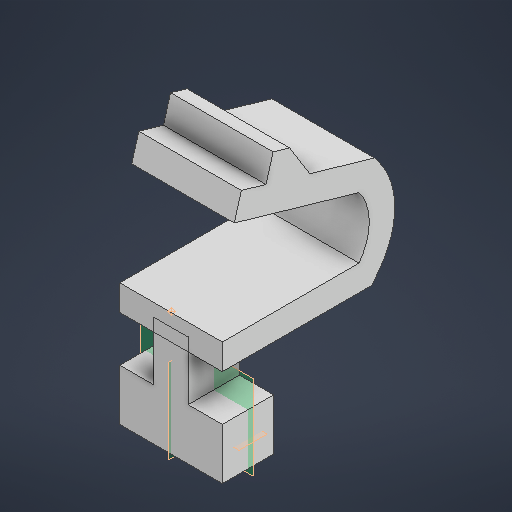
# Autodesk Inventor part: Clipper
Saved by Autodesk Inventor 2027 (Build 310192000, 192)
## iProperties
Created: 2026-03-31
Part Number: Clipper
Material: Generisch
Document SubType Name: Modeling
Designer: thomas
Density: 1 g/cm^3
Appearance: Vorgabe
Author: thomas
Autodesk Inventor part; units mm, degrees
ref_plane "YZ Plane" through (0, 0, 0) normal (1, 0, 0) x (0, 1, 0)
ref_plane "XZ Plane" through (0, 0, 0) normal (0, 1, 0) x (-1, 0, 0)
ref_plane "XY Plane" through (0, 0, 0) normal (0, 0, 1) x (1, 0, 0)
sketch "Sketch6" plane through (0, 0, 0) normal (0, 0, 1) x (1, 0, 0)
  line L0 (3, -1.5) -> (3, 1.5)
  line L1 (3, 1.5) -> (-3, 1.5)
  line L2 (-3, 1.5) -> (-3, -1.5)
  line L3 (-3, -1.5) -> (3, -1.5)
  line L4 (3, -1.5) -> (-3, 1.5) construction
  line L5 (3, 1.5) -> (-3, -1.5) construction
  point P0 (0, 0)
  dimension "d11" = 3
  dimension "d12" = 6
  constraints: 12 end point, 2 midpoint, 2 parallel, 1 perpendicular, 1 vertical
  measures "d11" distance of L0.start L0.end
  measures "d12" distance of L1.end L0.end
extrude "Extrusion4" add sketch "Sketch6" along normal mid plane 3
ref_plane "Work Plane1" through (0, 0, 0) normal (0, 0, 1) x (1, 0, 0)
sketch "Sketch8" plane through (0, 0, 1.5) normal (0, 0, 1) x (1, 0, 0)
  line L0 (-1, -1.5) -> (-1, 1.5)
  line L1 (-1, 1.5) -> (1, 1.5)
  line L2 (1, 1.5) -> (1, -1.5)
  line L3 (1, -1.5) -> (-1, -1.5)
  line L4 (-1, -1.5) -> (1, 1.5) construction
  line L5 (-1, 1.5) -> (1, -1.5) construction
  line L6 (3, 1.5) -> (-3, 1.5) projected
  point P0 (0, 0)
  dimension "d19" = 3
  dimension "d20" = 2
  constraints: 12 end point, 2 midpoint, 2 parallel, 1 collinear, 1 perpendicular
  measures "d19" distance of L0.start L0.end
  measures "d20" distance of L0.end L1.end
extrude "Extrusion6" add sketch "Sketch8" along normal blind 1.5
ref_plane "Work Plane4" through (-3, 0, -1.5) normal (0, 1, 0) x (1, 0, 0)
ref_plane "Work Plane5" through (0, -1.5, 1.5) normal (-1, 0, 0) x (0, 0, 1)
sketch "Sketch9" plane through (0, 0, 3) normal (0, 0, 1) x (1, 0, 0)
  point P0 (0, 0)
sketch "Sketch10" plane through (0, -1.5, 1.5) normal (-1, 0, 0) x (0, 0, 1)
  point P0 (-1.5, 1.5)
sketch "Sketch11" plane through (0, 0, 3) normal (0, 0, 1) x (1, 0, 0)
  point P0 (0, 0)
sketch "Sketch12" plane through (0, -1.5, 1.5) normal (-1, 0, 0) x (0, 0, 1)
  point P0 (-1.5, 1.5)
sketch "Sketch13" plane through (0, -1.5, 1.5) normal (-1, 0, 0) x (0, 0, 1)
  point P0 (-1.5, 1.5)
sketch "Sketch15" plane through (0, -1.5, 1.5) normal (-1, 0, 0) x (0, 0, 1)
  line L0 (4.175, 0) -> (4.175, 8)
  arc A0 (7.75, 8) -> (4.175, 8) centre (5.9625, 5.5907) ccw
  line L1 (7.75, 8) -> (9.858, 0.6982)
  line L2 (0, 0) -> (1.5, 0) projected
  line L3 (1.5, 0) -> (6.1638, 0) construction
  line L4 (1.5, 3) -> (1.5, 0) projected
  point P0 (-1.5, 1.5)
  dimension "d31" = 8
  dimension "d34" = 7.6
  dimension "d41" = 2.675
  dimension "d48" = 3.575
  constraints: 6 end point, 2 point on circle, 1 centre point, 1 horizontal, 1 point on line, 1 vertical
  measures "d31" distance of L0.start L0.end
  measures "d34" distance of L1.start L1.end
  measures "d41" distance between parallel lines of L0 L4
  measures "d48" distance of L1.start L0.end
sketch "Sketch18" plane through (-3, -1.5, -1.5) normal (0, -1, 0) x (1, 0, 0)
  line L0 (6, 5.675) -> (0, 5.675)
  line L1 (0, 5.675) -> (0, 7.175)
  line L2 (0, 7.175) -> (6, 7.175)
  line L3 (6, 7.175) -> (6, 5.675)
  line L4 (6, 5.675) -> (0.1205, 6.5404) construction
  line L5 (0, 5.675) -> (6, 7.175) construction
  line L6 (2, 4.5) -> (4, 4.5) projected
  point P0 (3, 1.5)
  point P1 (2.2234, 6.2309)
  point P2 (3, 4.5)
  point P3 (3, 4.5)
  point P4 (3, 7.175)
  point P5 (3, 7.175)
  dimension "d37" = 6
  dimension "d38" = 1.5
  dimension "d42" = 0
  constraints: 12 end point, 2 midpoint, 2 parallel, 2 point on line, 1 coincident, 1 horizontal, 1 perpendicular
  measures "d37" distance of L0.start L0.end
  measures "d38" distance of L0.end L1.end
  measures "d42" distance of point (3, 4.5) point (3, 4.5)
sweep "Sweep1" add profiles "Sketch18" path "Sketch15" separate body path curves L0 A0 L1
sketch "Sketch19" plane through (-3, 7.7899, 10.4389) normal (0, 0.2773708, 0.9607629) x (1, 0, 0)
  line L0 (0, -7.604) -> (0, 0.0821) projected
  line L1 (6, -0.9095) -> (6, -8.5095) projected
  line L2 (0, -6.0095) -> (6, -6.0095)
  line L3 (6, -6.0095) -> (6, -7.0095)
  line L4 (6, -7.0095) -> (0, -7.0095)
  line L5 (0, -7.0095) -> (0, -6.0095)
  line L6 (6, -8.5095) -> (0, -8.5095) projected
  point P0 (3, -4.5888)
  point P1 (0, -7.0095)
  point P2 (6, -6.0095)
  point P3 (0, -7.0095)
  dimension "d49" = 1.5
  dimension "d50" = 1
  constraints: 8 end point, 2 parallel, 2 point on line, 1 horizontal, 1 perpendicular
  measures "d49" distance between parallel lines of L6 L4
  measures "d50" distance between parallel lines of L4 L2
extrude "Extrusion7" add sketch "Sketch19" along normal blind 1.5 bodies 2
sketch "Sketch20" plane through (-3, -1.5, 4.175) normal (-1, 0, 0) x (0, 0, 1)
  line L0 (7.9307, 3.5162) -> (9.3719, 3.9322) projected
  line L1 (9.3719, 3.9322) -> (7.4684, 5.1177)
  line L2 (7.9307, 3.5162) -> (6.3756, 8.9028) projected
  point P0 (-4.175, 1.5)
  constraints: 2 end point, 1 point on line
extrude "Extrusion8" add sketch "Sketch20" against normal blind 6 bodies 2
sketch "Sketch21" plane through (0, 0, 3) normal (0, 0, 1) x (1, 0, 0)
  line L0 (-1, 1.5) -> (-3, 1.5) projected
  line L1 (1, -1.5) -> (1, 1.5) projected
  line L2 (-1, 1.5) -> (1, 1.5)
  line L3 (1, 1.5) -> (1, -1.5)
  line L4 (1, -1.5) -> (-1, -1.5)
  line L5 (-1, -1.5) -> (-1, 1.5)
  point P0 (0, 0)
  constraints: 8 end point, 2 parallel, 1 horizontal, 1 perpendicular
extrude "Extrusion9" add sketch "Sketch21" along normal blind 1.925 bodies 1
equation "\"d11\" = PCB_thickness"
equation "\"d12\" = clipper_uppter_t_length"
equation "\"d13\" = 0.5 * wall_thickness"
equation "\"d19\" = PCB_thickness"
equation "\"d20\" = clipp_lower_t_part_thickness"
equation "\"d21\" = 0.25 * wall_thickness"
equation "\"d31\" = arm_heigth"
equation "\"d34\" = 0.95 * arm_heigth"
equation "\"d41\" = 0.5 * spring_thickness + 0.35 * gap_width"
equation "\"d48\" = 0.65 * gap_width"
equation "\"d37\" = spring_width"
equation "\"d38\" = spring_thickness"
equation "\"d49\" = hook_offset"
equation "\"d46\" = spring_width"
equation "\"d51\" = 0.35 * gap_width"
equation "\"wall_thickness\" = 6"
equation "\"PCB_thickness\" = 3"
equation "\"clipp_lower_t_part_thickness\" = 2"
equation "\"clipper_uppter_t_length\" = 6"
equation "\"arm_heigth\" = 8"
equation "\"arc_radius\" = 1.3"
equation "\"gap_width\" = 5.5"
equation "\"spring_thickness\" = 1.5"
equation "\"spring_width\" = 6"
equation "\"hook_length\" = 3"
equation "\"hook_offset\" = 1.5"
body "Solid3"
body "Solid4"
